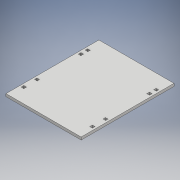
# Autodesk Inventor part: P3
Saved by Autodesk Inventor 2018 (Build 220112000, 112)
## iProperties
Created: 2018-02-28
Part Number: P3
Material: Generic
Document SubType Name: Modeling
Designer: isai
Density: 1 g/cm^3
Appearance: Default
Author: isai
Autodesk Inventor part; units mm, degrees
ref_plane "YZ Plane" through (0, 0, 0) normal (1, 0, 0) x (0, 1, 0)
ref_plane "XZ Plane" through (0, 0, 0) normal (0, 1, 0) x (-1, 0, 0)
sketch "Sketch1" plane through (0, 0, 0) normal (0, 0, 1) x (1, 0, 0)
  line L0 (0, -20) -> (0, 0)
  line L1 (0, -96.4) -> (0, -23.6)
  line L2 (4, -23.6) -> (0, -23.6)
  line L3 (0, -20) -> (4, -20)
  line L4 (4, 0) -> (0, 0)
  line L5 (0, -140) -> (0, -100)
  line L6 (0, -96.4) -> (4, -96.4)
  line L7 (4, -100) -> (0, -100)
  line L8 (4, -140) -> (0, -140)
  line L9 (107.2, -23.6) -> (107.2, -96.4)
  line L10 (107.2, -100) -> (107.2, -140)
  line L11 (107.2, -100) -> (103.2, -100)
  line L12 (103.2, -96.4) -> (107.2, -96.4)
  line L13 (103.2, -140) -> (107.2, -140)
  line L14 (103.2, -20) -> (107.2, -20)
  line L15 (107.2, 0) -> (107.2, -20)
  line L16 (103.2, 0) -> (107.2, 0)
  line L17 (4, 0) -> (103.2, 0)
  line L18 (4, -140) -> (103.2, -140)
  line L19 (0, -20) -> (4, -20)
  line L20 (4, -20) -> (4, -23.6)
  line L21 (4, -23.6) -> (0, -23.6)
  line L22 (0, -23.6) -> (0, -20)
  line L23 (0, -96.4) -> (4, -96.4)
  line L24 (4, -96.4) -> (4, -100)
  line L25 (4, -100) -> (0, -100)
  line L26 (0, -100) -> (0, -96.4)
  line L27 (103.2, -96.4) -> (107.2, -96.4)
  line L28 (107.2, -96.4) -> (107.2, -100)
  line L29 (107.2, -100) -> (103.2, -100)
  line L30 (103.2, -100) -> (103.2, -96.4)
  line L31 (103.2, -20) -> (107.2, -20)
  line L32 (107.2, -20) -> (107.2, -23.6)
  line L33 (107.2, -23.6) -> (103.2, -23.6)
  line L34 (103.2, -23.6) -> (103.2, -20)
  line L35 (0, 0) -> (-3, 0)
  line L36 (-3, 0) -> (-3, -140)
  line L37 (-3, -140) -> (0, -140)
  line L38 (0, -140) -> (0, 0)
  line L39 (107.2, 0) -> (110.2, 0)
  line L40 (110.2, 0) -> (110.2, -140)
  line L41 (110.2, -140) -> (107.2, -140)
  line L42 (107.2, -140) -> (107.2, 0)
  point P0 (0, 0)
  dimension "d0" = 3
  dimension "d1" = 3
  constraints: 86 end point, 13 parallel, 7 horizontal, 6 perpendicular, 1 point on line
  measures "d0" distance of L37.end L36.end
  measures "d1" distance of L40.end L41.end
extrude "Extrusion1" add sketch "Sketch1" along normal blind 4 contours L22 L1 L26 L5 L37 L36 L35 L0 | L0 L4 L17 L16 L15 L14 L34 L33 L9 L12 L30 L11 L10 L13 L18 L8 L5 L7 L24 L6 L1 L2 L20 L3 | L39 L40 L41 L10 L28 L9 L32 L15
sketch "Sketch2" plane through (0, 0, 4) normal (0, 0, 1) x (1, 0, 0)
  line L0 (107.2, -20) -> (107.2, -23.6) projected
  line L1 (107.2, -23.6) -> (103.2, -23.6) projected
  line L2 (103.2, -23.6) -> (103.2, -20) projected
  line L3 (103.2, -20) -> (107.2, -20) projected
  line L4 (107.2, -96.4) -> (107.2, -100) projected
  line L5 (107.2, -100) -> (103.2, -100) projected
  line L6 (103.2, -100) -> (103.2, -96.4) projected
  line L7 (103.2, -96.4) -> (107.2, -96.4) projected
  line L8 (0, -96.4) -> (4, -96.4) projected
  line L9 (4, -96.4) -> (4, -100) projected
  line L10 (4, -100) -> (0, -100) projected
  line L11 (0, -100) -> (0, -96.4) projected
  line L12 (0, -23.6) -> (0, -20) projected
  line L13 (0, -20) -> (4, -20) projected
  line L14 (4, -20) -> (4, -23.6) projected
  line L15 (4, -23.6) -> (0, -23.6) projected
  line L16 (110.2, 0) -> (-3, 0) projected
  line L17 (-3, 0) -> (-3, -140) projected
  line L18 (-3, -140) -> (110.2, -140) projected
  line L19 (110.2, -140) -> (110.2, 0) projected
  line L20 (107.2, -120) -> (103.2, -120)
  line L21 (103.2, -120) -> (103.2, -116)
  line L22 (103.2, -116) -> (107.2, -116)
  line L23 (107.2, -116) -> (107.2, -120)
  line L24 (107.2, -120) -> (103.2, -116) construction
  line L25 (103.2, -120) -> (107.2, -116) construction
  line L26 (107.2, -34) -> (103.2, -34)
  line L27 (103.2, -34) -> (103.2, -30)
  line L28 (103.2, -30) -> (107.2, -30)
  line L29 (107.2, -30) -> (107.2, -34)
  line L30 (107.2, -34) -> (103.2, -30) construction
  line L31 (103.2, -34) -> (107.2, -30) construction
  point P0 (0, 0)
  point P1 (105.2, -118)
  point P2 (105.2, -32)
  dimension "d4" = 4
  dimension "d5" = 20
  dimension "d6" = 4
  dimension "d7" = 4
  dimension "d8" = 30
  constraints: 24 end point, 4 midpoint, 4 parallel, 2 horizontal, 2 perpendicular
  measures "d4" distance of L20.end L21.end
  measures "d5" distance between parallel lines of L18 L20
  measures "d6" distance of L27.end L28.end
  measures "d7" distance of L26.end L27.end
  measures "d8" distance between parallel lines of L28 L16
extrude "Extrusion2" cut sketch "Sketch2" against normal blind 10 contours L20 L21 L22 L23 | L26 L27 L28 L29
ref_plane "Work Plane1" through (53.6, -140, 0) normal (1, 0, 0) x (0, 0, -1)
mirror "Mirror1" about plane through (53.6, -140, 0) normal (1, 0, 0) of "Extrusion2"
body "Solid1"
